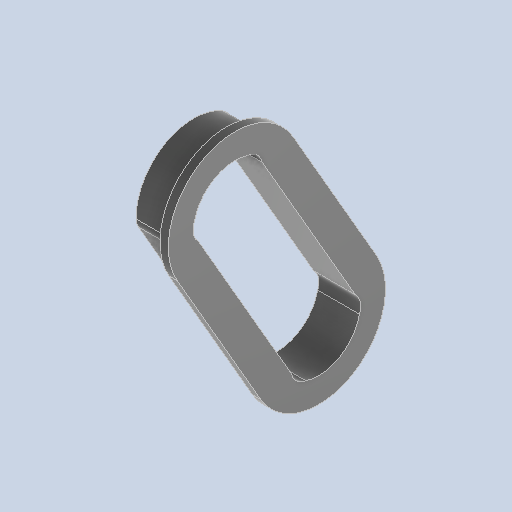
# Autodesk Inventor part: SliderProtectionFrame
Saved by Autodesk Inventor 2024.2 (Build 282272000, 272)
## iProperties
Created: 2024-01-06
Part Number: SliderProtectionFrame
Material: Acetal Resin, Black
Document SubType Name: Modeling
Designer: Masato Kubotera
Density: 1.425 g/cm^3
Appearance: Smooth - Black
Mass: 1.19185 g
Surface Area: 13.1636 cm^2
Volume: 0.836385 cm^3
Vendor: meviy
Author: Masato Kubotera
Autodesk Inventor part; units mm, degrees
ref_plane "YZ Plane" through (0, 0, 0) normal (1, 0, 0) x (0, 1, 0)
ref_plane "XZ Plane" through (0, 0, 0) normal (0, 1, 0) x (-1, 0, 0)
ref_plane "XY Plane" through (0, 0, 0) normal (0, 0, 1) x (1, 0, 0)
derived "LegLinkBasis.ipt"
sketch "Sketch1" plane through (0, 0, 0) normal (0, 1, 0) x (-1, 0, 0)
  line L0 (-32, 15) -> (-32, 0) construction
  line L1 (-32, 0) -> (0, 0) construction
  arc A0 (-4.9497, -4.9497) -> (6.7615, 1.8117) centre (0, 0) ccw
  line L2 (0, 0) -> (0, -25) construction
  line L3 (1.023, 23.2282) -> (-45.6223, 104.0202)
  line L4 (-66.25, 114.7484) -> (0, 0) construction
  line L5 (6.7615, 1.8117) -> (1.023, 23.2282)
  line L6 (-22.2997, 63.6242) -> (-43.9503, 51.1242) construction
  line L7 (-61.3003, 119.6981) -> (-45.6223, 104.0202)
  arc A1 (-61.3003, 119.6981) -> (-73.0115, 112.9366) centre (-66.25, 114.7484) ccw
  line L8 (-20.6277, 10.7282) -> (-67.273, 91.5202)
  line L9 (-4.9497, -4.9497) -> (-20.6277, 10.7282)
  line L10 (-73.0115, 112.9366) -> (-67.273, 91.5202)
  line L11 (-78.1154, 64.8742) -> (-58.4455, 76.2306) construction
  line L12 (-26.1899, 20.3622) -> (-90.7012, 132.099)
  line L13 (-32, 15) -> (-98.25, 129.7484) construction
  line L14 (-26.1899, 20.3622) -> (-25.2385, 16.8117)
  arc A2 (-36.9497, 10.0503) -> (-25.2385, 16.8117) centre (-32, 15) ccw
  arc A3 (-93.3003, 134.6981) -> (-105.0115, 127.9366) centre (-98.25, 129.7484) ccw
  line L15 (-90.7012, 132.099) -> (-93.3003, 134.6981)
  circle A4 centre (-10, 17.3205) radius 20 construction
  circle A5 centre (0, 0) radius 40 construction
  line L16 (0, 0) -> (10, 17.3205) construction
  line L17 (10, 17.3205) -> (20, 34.641) construction
  arc A6 (-15.9891, 40.194) -> (-26.8144, 33.944) centre (-20, 34.641) ccw
  line L18 (-26.8144, 33.944) -> (-14.0109, 11.7675)
  line L19 (-20.4127, 22.8558) -> (-9.5873, 29.1058) construction
  line L20 (-15.9891, 40.194) -> (-3.1856, 18.0175)
  arc A7 (-14.0109, 11.7675) -> (-3.1856, 18.0175) centre (-10, 17.3205) ccw
  arc A8 (-17.3769, 38.8977) -> (-24.9979, 34.4977) centre (-20, 34.641) ccw construction
  line L21 (-24.9979, 34.4977) -> (-12.6231, 13.0638) construction
  line L22 (-17.3769, 38.8977) -> (-5.0021, 17.4638) construction
  arc A9 (-12.6231, 13.0638) -> (-5.0021, 17.4638) centre (-10, 17.3205) ccw construction
  line L23 (-86.9103, 90.1073) -> (-82.5801, 92.6073) construction
  line L24 (-82.5801, 92.6073) -> (-65.0801, 62.2965) construction
  line L25 (-65.0801, 62.2965) -> (-69.4103, 59.7965) construction
  line L26 (-69.4103, 59.7965) -> (-86.9103, 90.1073) construction
  line L27 (-86.9103, 90.1073) -> (-65.0801, 62.2965) construction
  line L28 (-82.5801, 92.6073) -> (-69.4103, 59.7965) construction
  line L29 (-82.4103, 82.3131) -> (-78.0801, 84.8131) construction
  line L30 (-78.1603, 74.9519) -> (-73.8301, 77.4519) construction
  line L31 (-69.5801, 70.0907) -> (-73.9103, 67.5907) construction
  line L32 (-69.5118, 70.0724) -> (-73.9286, 67.5224)
  line L33 (-73.9286, 67.5224) -> (-82.4786, 82.3314)
  line L34 (-82.4786, 82.3314) -> (-78.0618, 84.8814)
  line L35 (-78.0618, 84.8814) -> (-69.5118, 70.0724)
  line L36 (-69.5118, 70.0724) -> (-82.4786, 82.3314) construction
  line L37 (-73.9286, 67.5224) -> (-78.0618, 84.8814) construction
  arc A10 (-82.4786, 82.3314) -> (-80.9786, 79.7333) centre (-81.7286, 81.0324) ccw
  arc A11 (-75.4286, 70.1205) -> (-73.9286, 67.5224) centre (-74.6786, 68.8214) ccw
  line L38 (-84.7452, 91.3573) -> (-67.2452, 61.0465) construction
  arc A12 (-76.5618, 82.2833) -> (-78.0618, 84.8814) centre (-77.3118, 83.5824) ccw
  arc A13 (-69.5118, 70.0724) -> (-71.0118, 72.6705) centre (-70.2618, 71.3714) ccw
  line L39 (-33.1578, 57.6439) -> (-28.8277, 60.1439) construction
  line L40 (-28.9262, 50.2144) -> (-33.0594, 67.5734) construction
  line L41 (-28.9262, 50.2144) -> (-37.4762, 65.0234)
  line L42 (-33.0594, 67.5734) -> (-24.5094, 52.7644)
  line L43 (-24.5094, 52.7644) -> (-37.4762, 65.0234) construction
  line L44 (-24.4078, 42.4884) -> (-41.9078, 72.7993) construction
  line L45 (-41.9078, 72.7993) -> (-20.0777, 44.9884) construction
  line L46 (-39.7428, 74.0493) -> (-22.2428, 43.7384) construction
  line L47 (-37.5777, 75.2993) -> (-24.4078, 42.4884) construction
  line L48 (-37.5777, 75.2993) -> (-20.0777, 44.9884) construction
  arc A14 (-30.4262, 52.8125) -> (-28.9262, 50.2144) centre (-29.6762, 51.5134) ccw
  arc A15 (-24.5094, 52.7644) -> (-26.0094, 55.3625) centre (-25.2594, 54.0634) ccw
  line L49 (-24.5777, 52.7827) -> (-28.9078, 50.2827) construction
  line L50 (-20.0777, 44.9884) -> (-24.4078, 42.4884) construction
  line L51 (-24.5094, 52.7644) -> (-28.9262, 50.2144)
  arc A16 (-31.5594, 64.9753) -> (-33.0594, 67.5734) centre (-32.3094, 66.2744) ccw
  line L52 (-37.4078, 65.0051) -> (-33.0777, 67.5051) construction
  arc A17 (-37.4762, 65.0234) -> (-35.9762, 62.4253) centre (-36.7262, 63.7244) ccw
  line L53 (-37.4762, 65.0234) -> (-33.0594, 67.5734)
  line L54 (-41.9078, 72.7993) -> (-37.5777, 75.2993) construction
  line L55 (-105.0115, 127.9366) -> (-96.773, 97.1901)
  line L56 (-96.773, 97.1901) -> (-59.4578, 32.5583)
  line L57 (-59.4578, 32.5583) -> (-36.9497, 10.0503)
  line L58 (-229.0113, 122.0356) -> (-99.9887, 122.0356) construction
  arc A18 (-96.4383, 122.9869) -> (-96.4383, 136.5098) centre (-98.25, 129.7484) ccw construction
  line L59 (-99.9887, 122.0356) -> (-96.4383, 122.9869) construction
  line L60 (-96.4383, 136.5098) -> (-127.1848, 144.7484) construction
  line L61 (-127.1848, 144.7484) -> (-201.8152, 144.7484) construction
  line L62 (-201.8152, 144.7484) -> (-232.5617, 136.5098) construction
  arc A19 (-232.5617, 136.5098) -> (-232.5617, 122.9869) centre (-230.75, 129.7484) ccw construction
  line L63 (-229.0113, 122.0356) -> (-232.5617, 122.9869) construction
  arc A20 (-64.4383, 107.9869) -> (-64.4383, 121.5098) centre (-66.25, 114.7484) ccw construction
  line L64 (-64.4383, 107.9869) -> (-85.8547, 102.2484) construction
  line L65 (-64.4383, 121.5098) -> (-85.8547, 127.2484) construction
  line L66 (-179.1453, 102.2484) -> (-85.8547, 102.2484) construction
  line L67 (-179.1453, 127.2484) -> (-85.8547, 127.2484) construction
  line L68 (-200.5617, 121.5098) -> (-179.1453, 127.2484) construction
  arc A21 (-200.5617, 121.5098) -> (-200.5617, 107.9869) centre (-198.75, 114.7484) ccw construction
  line L69 (-200.5617, 107.9869) -> (-179.1453, 102.2484) construction
  arc A22 (-181.5536, 120.9984) -> (-181.5536, 108.4984) centre (-178.75, 114.7484) ccw construction
  line L70 (-155.9464, 108.4984) -> (-181.5536, 108.4984) construction
  line L71 (-155.9464, 120.9984) -> (-181.5536, 120.9984) construction
  arc A23 (-155.9464, 108.4984) -> (-155.9464, 120.9984) centre (-158.75, 114.7484) ccw construction
  line L72 (-179.1453, 127.2484) -> (-198.5998, 122.0356)
  line L73 (-179.1453, 127.2484) -> (-158.3547, 127.2484)
  line L74 (-168.75, 120.9984) -> (-168.75, 108.4984) construction
  line L75 (-158.3547, 127.2484) -> (-138.9002, 122.0356)
  line L76 (-138.9002, 122.0356) -> (-99.9887, 122.0356)
  line L77 (-99.9887, 122.0356) -> (-80.5342, 127.2484)
  line L78 (-31.023, 28.7333) -> (-36.2358, 48.1878)
  line L79 (-36.2358, 48.1878) -> (-55.6915, 81.8862)
  line L80 (-55.6915, 81.8862) -> (-69.9332, 96.1279)
  line L81 (-66.0326, 78.9462) -> (-71.2454, 98.4006)
  line L82 (-55.6373, 60.941) -> (-66.0326, 78.9462)
  line L83 (-55.6373, 60.941) -> (-41.3956, 46.6993)
  line L84 (-55.6915, 81.8862) -> (-72.4858, 110.9747)
  point P0 (-75.9952, 76.2019)
  point P1 (-83.2452, 88.7593)
  point P2 (-68.7452, 63.6445)
  point P3 (-30.9928, 58.8939)
  point P4 (-38.2428, 71.4513)
  point P5 (-23.7428, 46.3365)
  point P6 (-164.5, 122.0356)
  point P7 (-164.5, 144.7484)
  point P8 (-132.5, 102.2484)
  point P9 (-132.5, 127.2484)
sketch "Sketch2" plane through (0, 0, 0) normal (0, 1, 0) x (-1, 0, 0)
  line L0 (-15.9891, 40.194) -> (-3.1856, 18.0175) projected
  arc A0 (-15.9891, 40.194) -> (-26.8144, 33.944) centre (-20, 34.641) ccw projected
  arc A1 (-17.3769, 38.8977) -> (-24.9979, 34.4977) centre (-20, 34.641) ccw projected
  line L1 (-17.3769, 38.8977) -> (-5.0021, 17.4638) projected
  line L2 (-26.8144, 33.944) -> (-14.0109, 11.7675) projected
  arc A2 (-14.0109, 11.7675) -> (-3.1856, 18.0175) centre (-10, 17.3205) ccw projected
  arc A3 (-12.6231, 13.0638) -> (-5.0021, 17.4638) centre (-10, 17.3205) ccw projected
  line L3 (-20.4127, 22.8558) -> (-9.5873, 29.1058) construction
  line L4 (-66.25, 114.7484) -> (0, 0) construction
  circle A4 centre (-10, 17.3205) radius 7 construction
  line L5 (1.023, 23.2282) -> (-45.6223, 104.0202) projected
  line L6 (-20.6277, 10.7282) -> (-67.273, 91.5202) projected
  arc A5 (-5.1148, 16.2553) -> (-5.6089, 18.515) centre (-6.9559, 17.0365) ccw
  line L7 (-24.9979, 34.4977) -> (-12.6231, 13.0638) projected
  arc A6 (-13.23, 14.115) -> (-11.5201, 12.5572) centre (-11.2761, 14.5422) ccw
  arc A7 (-16.77, 37.8465) -> (-18.4799, 39.4043) centre (-18.7239, 37.4193) ccw
  arc A8 (-24.8852, 35.7062) -> (-24.3911, 33.4465) centre (-23.0441, 34.925) ccw
  arc A9 (-16.9282, 13.3205) -> (-3.0718, 21.3205) centre (-10, 17.3205) ccw
  line L8 (-3.0718, 21.3205) -> (-13.0718, 38.641)
  line L9 (-16.9282, 13.3205) -> (-26.9282, 30.641)
  arc A10 (-13.0718, 38.641) -> (-26.9282, 30.641) centre (-20, 34.641) ccw
  point P0 (-24.3911, 33.4465)
  point P1 (-24.8852, 35.7062)
  point P2 (-18.4799, 39.4043)
  point P3 (-16.77, 37.8465)
  point P4 (-11.5201, 12.5572)
  point P5 (-13.23, 14.115)
  point P6 (-16.9282, 13.3205)
  dimension "d1" = 14
  dimension "d2" = 2
  dimension "d5" = 1
  constraints: 14 point on circle, 14 symmetric about line, 7 centre point, 4 end point, 2 coincident, 1 parallel, 1 point on line, 1 tangent, 4 other
  measures "d1" diameter of A4
  measures "d2" radius of A5
  measures "d5" radial gap between concentric circles of A9 A4
extrude "Extrusion1" add sketch "Sketch2" along normal blind 5 contours L0 A2 L2 A0 | L9 A10 L8 A9
extrude "Extrusion2" cut sketch "Sketch2" along normal blind 4 contours L9 A10 L8 A9
fillet "Fillet1" radius 2 4 edges at (15.9891, 2, 40.194) (26.8144, 2, 33.944) (3.1856, 2, 18.0175) (14.0109, 2, 11.7675)
body "Solid1"
